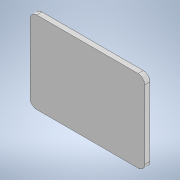
# Autodesk Inventor part: pcb_placeholder_larger
Saved by Autodesk Inventor 2020.2 (Build 242310000, 310)
## iProperties
Created: 2020-09-26
Part Number: pcb_placeholder_larger
Material: Generic
Document SubType Name: Modeling
Designer: Krishna Makhija
Density: 1 g/cm^3
Appearance: Default
Author: Krishna Makhija
Autodesk Inventor part; units mm, degrees
ref_plane "YZ Plane" through (0, 0, 0) normal (1, 0, 0) x (0, 1, 0)
ref_plane "XZ Plane" through (0, 0, 0) normal (0, 1, 0) x (-1, 0, 0)
ref_plane "XY Plane" through (0, 0, 0) normal (0, 0, 1) x (1, 0, 0)
sketch "Sketch3" plane through (0, 0, 0) normal (0, 0, 1) x (1, 0, 0)
  line L0 (17.4998, -12.4998) -> (-17.4998, -12.4998)
  line L1 (-17.4998, -12.4998) -> (-17.4998, 12.4998)
  line L2 (-17.4998, 12.4998) -> (17.4998, 12.4998)
  line L3 (17.4998, 12.4998) -> (17.4998, -12.4998)
  line L4 (17.4998, -12.4998) -> (-17.4998, 12.4998) construction
  line L5 (-17.4998, -12.4998) -> (17.4998, 12.4998) construction
  point P0 (0, 0)
  constraints: 12 end point, 2 midpoint, 2 parallel, 1 horizontal, 1 perpendicular
extrude "Extrusion2" add sketch "Sketch3" along normal blind 1.6
fillet "Fillet2" radius 2 4 edges at (-17.4998, -12.4998, 0.8) (17.4998, -12.4998, 0.8) (17.4998, 12.4998, 0.8) (-17.4998, 12.4998, 0.8)
body "Solid2"
